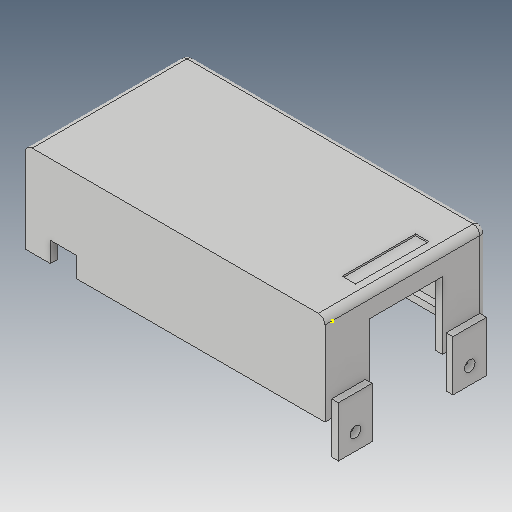
# Autodesk Inventor part: sideboard_top
Saved by Autodesk Inventor 2019 (Build 230136000, 136)
## iProperties
Created: 2020-05-11
Part Number: sideboard_top
Material: Generic
Document SubType Name: Modeling
Designer: Mateusz
Density: 1 g/cm^3
Appearance: Default
Author: Mateusz
Autodesk Inventor part; units mm, degrees
ref_plane "YZ Plane" through (0, 0, 0) normal (1, 0, 0) x (0, 1, 0)
ref_plane "XZ Plane" through (0, 0, 0) normal (0, 1, 0) x (-1, 0, 0)
ref_plane "XY Plane" through (0, 0, 0) normal (0, 0, 1) x (1, 0, 0)
sketch "Sketch1" plane through (0, 0, 0) normal (0, 1, 0) x (-1, 0, 0)
  line L0 (0, 0) -> (0, -44)
  line L1 (0, -44) -> (85, -44)
  line L2 (85, -44) -> (85, 0)
  line L3 (85, 0) -> (0, 0)
  line L4 (0, -46) -> (-2, -46)
  line L5 (-2, -46) -> (-2, 0)
  line L6 (-2, 0) -> (-2, 2)
  line L7 (-2, 2) -> (85, 2)
  line L8 (85, 2) -> (87, 2)
  line L9 (87, 2) -> (87, -46)
  line L10 (87, -46) -> (0, -46)
  dimension "d0" = 44
  dimension "d2" = 2
  dimension "d3" = 2
  dimension "d4" = 2
  dimension "d5" = 2
  constraints: 22 end point, 7 perpendicular, 6 point on line, 1 vertical
  measures "d0" distance of L0.start L0.end
  measures "d2" distance of L0.end L4.start
  measures "d3" distance of L4.start L4.end
  measures "d4" distance of L5.end L6.end
  measures "d5" distance of L7.end L8.end
extrude "Extrusion1" add sketch "Sketch1" along normal blind 2 contours L3 L2 L1 L0 | L4 L5 L6 L7 L8 L9 L10
extrude "Extrusion2" add sketch "Sketch1" against normal blind 25
sketch "Sketch2" plane through (2, 2, 2) normal (1, 0, 0) x (0, 0, -1)
  point P0 (2, -2)
sketch "Sketch3" plane through (2, 2, 2) normal (1, 0, 0) x (0, 0, -1)
  line L0 (0, -27) -> (13.1, -27)
  line L1 (46, -27) -> (2, -27) projected
  line L2 (0, -27) -> (48, -27) projected
  line L3 (48, -27) -> (34.9, -27)
  line L4 (34.9, -27) -> (34.9, -7)
  line L5 (34.9, -7) -> (13.1, -7)
  line L6 (13.1, -7) -> (13.1, -27)
  line L7 (13.1, -27) -> (34.9, -27)
  point P0 (2, -2)
  dimension "d10" = 13.1
  dimension "d11" = 13.1
  dimension "d12" = 20
  constraints: 12 end point, 3 perpendicular, 2 point on line, 1 collinear
  measures "d10" distance of L0.start L0.end
  measures "d11" distance of L2.end L3.end
  measures "d12" distance of L3.end L4.end
extrude "Extrusion3" cut sketch "Sketch3" against normal blind 25
fillet "Fillet1" radius 2 5 edges at (-42.5, 2, -46) (2, -11.5, -46) (2, 2, -22) (-87, 2, -22) (-87, -11.5, -46)
sketch "Sketch4" plane through (-87, -25, 2) normal (0, 0, 1) x (1, 0, 0)
  line L0 (2, 0) -> (0, 0) projected
  line L1 (0, 0) -> (7.4, 0)
  line L2 (87, 0) -> (2, 0) projected
  line L3 (7.4, 0) -> (15.2, 0)
  line L4 (15.2, 0) -> (15.2, 6)
  line L5 (15.2, 6) -> (7.4, 6)
  line L6 (7.4, 6) -> (7.4, 0)
  point P0 (87, 25)
  dimension "d16" = 7.4
  dimension "d17" = 7.8
  dimension "d18" = 6
  constraints: 10 end point, 2 perpendicular, 2 point on line, 1 vertical
  measures "d16" distance of L0.end L1.end
  measures "d17" distance of L1.end L3.end
  measures "d18" distance of L3.end L4.end
extrude "Extrusion4" cut sketch "Sketch4" against normal blind 25
sketch "Sketch5" plane through (0, 2, 0) normal (0, 1, 0) x (1, 0, 0)
  line L0 (2, 32.9) -> (0, 32.9) projected
  line L1 (0, 11.1) -> (2, 11.1) projected
  line L2 (0, 32.9) -> (0, 11.1)
  line L3 (0, 11.1) -> (-2, 11.1)
  line L4 (-2, 11.1) -> (-6, 11.1)
  line L5 (-6, 11.1) -> (-6, 32.9)
  line L6 (-6, 32.9) -> (-2, 32.9)
  line L7 (-2, 32.9) -> (-2, 11.1)
  point P0 (0, 0)
  dimension "d21" = 2
  dimension "d22" = 4
  dimension "d23" = 4
  constraints: 12 end point, 4 perpendicular, 1 point on line
  measures "d21" distance of L1.start L3.end
  measures "d22" distance of L3.end L4.end
  measures "d23" distance of L5.end L6.end
extrude "Extrusion5" cut sketch "Sketch5" against normal blind 0.5
sketch "Sketch6" plane through (-87, -25, -44) normal (-1, 0, 0) x (0, 0, 1)
  line L0 (46, 25) -> (0, 25) projected
  line L1 (23, 25) -> (23, 0)
  line L2 (46, 0) -> (0, 0) projected
  line L3 (23, 0) -> (28, 0)
  line L4 (28, 0) -> (28, 5)
  line L5 (28, 5) -> (18, 5)
  line L6 (18, 5) -> (18, 0)
  line L7 (23, 0) -> (18, 0)
  point P0 (44, 25)
  dimension "d26" = 5
  dimension "d27" = 5
  dimension "d28" = 10
  constraints: 12 end point, 3 perpendicular, 2 midpoint, 2 point on line, 1 collinear
  measures "d26" distance of L1.end L3.end
  measures "d27" distance of L3.end L4.end
  measures "d28" distance of L4.end L5.end
extrude "Extrusion6" add sketch "Sketch6" along normal blind 2
sketch "Sketch7" plane through (0, -25, 0) normal (0, -1, 0) x (1, 0, 0)
  line L0 (-87, -44) -> (-87, 2) projected
  line L1 (-87, -26) -> (-89, -26) projected
  line L2 (-87, -15.9645) -> (-87, -26)
  line L3 (-87, -26) -> (-89, -26)
  line L4 (-89, -26) -> (-89, -16) projected
  line L5 (-89, -26) -> (-89, -16)
  line L6 (-87, -16) -> (-89, -16) projected
  line L7 (-89, -16) -> (-87, -16)
  point P0 (0, 0)
  constraints: 8 end point, 2 collinear, 1 perpendicular, 1 point on line, 1 vertical
extrude "Extrusion7" add sketch "Sketch7" along normal blind 10
sketch "Sketch8" plane through (-89, -25, -44) normal (-1, 0, 0) x (0, 0, 1)
  line L0 (28, 0) -> (18, 0) projected
  line L1 (18, 0) -> (23, 0)
  line L2 (23, 0) -> (23, -5)
  circle A0 centre (23, -5) radius 1.6
  point P0 (44, 25)
  dimension "d33" = 5
  dimension "d34" = 3.2
  constraints: 4 end point, 1 centre point, 1 coincident, 1 midpoint, 1 perpendicular
  measures "d33" distance of L1.end L2.end
  measures "d34" diameter of A0
extrude "Extrusion8" cut sketch "Sketch8" against normal blind 10
sketch "Sketch9" plane through (2, -25, -11.1) normal (1, 0, 0) x (0, 0, -1)
  line L0 (-13.1, 0) -> (4.9, 0) projected
  line L1 (-13.1, 0) -> (-11.1, 0)
  line L2 (-11.1, 0) -> (-11.1, 5)
  line L3 (-11.1, 6) -> (-11.1, 0) projected
  line L4 (-11.1, 5) -> (-1.1, 5)
  line L5 (-1.1, 5) -> (-1.1, 0)
  line L6 (-1.1, 0) -> (-11.1, 0)
  line L7 (32.9, 0) -> (-11.1, 0) projected
  line L8 (32.9, 0) -> (32.9, 5)
  line L9 (32.9, 0) -> (32.9, 25) projected
  line L10 (32.9, 5) -> (22.9, 5)
  line L11 (22.9, 5) -> (22.9, 0)
  line L12 (22.9, 0) -> (32.9, 0)
  point P0 (-11.1, 25)
  dimension "d37" = 2
  dimension "d38" = 5
  dimension "d39" = 10
  dimension "d40" = 5
  dimension "d41" = 10
  constraints: 18 end point, 4 perpendicular, 4 point on line, 1 collinear, 1 horizontal
  measures "d37" distance of L0.start L1.end
  measures "d38" distance of L1.end L2.end
  measures "d39" distance of L2.end L4.end
  measures "d40" distance of L7.start L8.end
  measures "d41" distance of L8.end L10.end
extrude "Extrusion9" add sketch "Sketch9" along normal blind 2
sketch "Sketch10" plane through (0, -25, 0) normal (0, -1, 0) x (1, 0, 0)
  line L0 (4, -10) -> (4, 0) projected
  line L1 (2, -10) -> (4, -10) projected
  line L2 (4, -10) -> (2, -10)
  line L3 (2, 0) -> (2, -10) projected
  line L4 (2, -10) -> (2, 0)
  line L5 (2, 0) -> (4, 0)
  line L6 (4, 0) -> (4, -10)
  line L7 (4, -44) -> (4, -34) projected
  line L8 (4, -34) -> (4, -44)
  line L9 (2, -44) -> (4, -44) projected
  line L10 (4, -44) -> (2, -44)
  line L11 (2, -44) -> (2, -34)
  line L12 (2, 2) -> (2, -44) projected
  line L13 (4, -34) -> (2, -34)
  point P0 (0, 0)
  constraints: 16 end point, 4 collinear, 3 perpendicular, 1 point on line
extrude "Extrusion10" add sketch "Sketch10" along normal blind 10
sketch "Sketch11" plane through (4, -25, -11.1) normal (1, 0, 0) x (0, 0, -1)
  line L0 (-1.1, -10) -> (-11.1, -10) projected
  line L1 (-6.1, -10) -> (-6.1, -5)
  line L2 (22.9, -10) -> (32.9, -10) projected
  line L3 (27.9, -10) -> (27.9, -5)
  circle A0 centre (-6.1, -5) radius 1.6
  circle A1 centre (27.9, -5) radius 1.6
  point P0 (-11.1, 25)
  dimension "d46" = 5
  dimension "d47" = 5
  dimension "d48" = 3.2
  dimension "d49" = 3.2
  constraints: 4 end point, 2 centre point, 2 coincident, 2 midpoint, 2 vertical
  measures "d46" distance of L1.start L1.end
  measures "d47" distance of L3.start L3.end
  measures "d48" diameter of A0
  measures "d49" diameter of A1
extrude "Extrusion11" cut sketch "Sketch11" against normal blind 10
sketch "Sketch12" plane through (0, 0, 0) normal (0, 0, -1) x (-1, 0, 0)
  line L0 (0, -5) -> (0, -25) projected
  line L1 (71.8, -19) -> (71.8, -25) projected
  line L2 (0, -25) -> (71.8, -25)
  line L3 (71.8, -25) -> (71.8, -23)
  line L4 (71.8, -23) -> (0, -23)
  line L5 (0, -23) -> (0, -25)
  point P0 (0, 0)
  dimension "d52" = 2
  constraints: 8 end point, 3 perpendicular, 1 point on line
  measures "d52" distance of L1.end L3.end
extrude "Extrusion12" add sketch "Sketch12" along normal blind 2
sketch "Sketch13" plane through (-85, 0, -44) normal (0, 0, 1) x (1, 0, 0)
  line L0 (87, -25) -> (13.2, -25) projected
  line L1 (13.2, -23) -> (85, -23) projected
  line L2 (13.2, -25) -> (13.2, -23)
  line L3 (13.2, -23) -> (85, -23)
  line L4 (85, -5) -> (85, -25) projected
  line L5 (85, -23) -> (85, -25)
  line L6 (85, -25) -> (13.2, -25)
  point P0 (85, 0)
  constraints: 8 end point, 2 collinear, 1 perpendicular, 1 vertical
extrude "Extrusion13" add sketch "Sketch13" along normal blind 2
body "Solid1"
